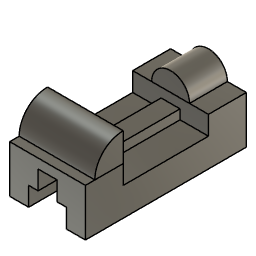
2 (Autodesk Fusion 360 design; units mm, degrees)
Autodesk Fusion 360 part; units mm, degrees
sketch "Sketch1" plane through (0, 0, 0) normal (0, 1, 0) x (1, 0, 0)
  line L0 (0, 0) -> (0, -50)
  line L1 (0, -50) -> (80, -50)
  line L2 (80, -50) -> (80, 0)
  line L3 (80, 0) -> (60, 0)
  line L4 (60, 0) -> (60, -20)
  line L5 (60, -20) -> (50, -20)
  line L6 (50, -20) -> (50, -40)
  line L7 (50, -40) -> (30, -40)
  line L8 (30, -40) -> (30, -20)
  line L9 (30, -20) -> (20, -20)
  line L10 (20, -20) -> (20, 0)
  line L11 (20, 0) -> (0, 0)
  dimension "d1" = 50
  constraint coincident L0.start L11.end
  constraint vertical L0
  constraint perpendicular L0 L1
  constraint perpendicular L1 L2
  constraint perpendicular L2 L3
  constraint perpendicular L3 L4
  constraint perpendicular L4 L5
  constraint perpendicular L3 L6
  constraint perpendicular L6 L7
  constraint perpendicular L7 L8
  constraint perpendicular L8 L9
  constraint perpendicular L9 L10
  constraint perpendicular L0 L11
  measures "d1" distance of L0.start L0.end
sketch "Sketch2" plane through (0, 0, 0) normal (0, 0, 1) x (1, 0, 0)
  line L0 (0, 0) -> (0, 170)
  line L1 (0, 170) -> (20, 170)
  line L2 (20, 170) -> (20, 0)
  line L3 (80, 0) -> (80, 170)
  line L4 (80, 170) -> (60, 170)
  line L5 (60, 170) -> (60, 0)
  dimension "d3" = 170
  constraint coincident L0.start origin
  constraint vertical L0
  constraint perpendicular L0 L1
  constraint perpendicular L1 L2
  constraint vertical L3
  constraint perpendicular L3 L4
  constraint perpendicular L4 L5
  measures "d3" distance of L0.start L0.end
sketch "Sketch3" plane through (0, 0, 0) normal (1, 0, 0) x (0, 1, 0)
  line L0 (0, 50) -> (10, 50)
  arc A0 (40, 80) -> (10, 50) centre (40, 50) ccw
  line L1 (40, 80) -> (40, 30)
  line L2 (40, 30) -> (130, 30)
  line L3 (130, 30) -> (130, 50)
  line L4 (130, 50) -> (170, 50)
  line L5 (170, 50) -> (170, 0)
  line L6 (130, 30) -> (170, 30)
  line L7 (10, 50) -> (40, 50)
  constraint horizontal L0
  constraint vertical L1
  constraint perpendicular L1 L2
  constraint perpendicular L2 L3
  constraint perpendicular L3 L4
  constraint perpendicular L4 L5
  constraint coincident L5 L6.end
  constraint perpendicular L5 L6
  constraint coincident A0.centre L7.end
  constraint perpendicular L1 L7
extrude "Extrude1" add sketch "Sketch1" along normal blind 40 makes body 1
sketch "Sketch5" plane through (0, 40, 0) normal (0, 1, 0) x (-1, 0, 0)
  line L0 (-20, 0) -> (0, 0)
  line L1 (0, 0) -> (0, 50)
  line L2 (0, 50) -> (-80, 50)
  line L3 (-80, 50) -> (-80, 0)
  line L4 (-80, 0) -> (-60, 0)
  line L5 (-60, 0) -> (-60, 20)
  line L6 (-60, 20) -> (-50, 20)
  line L7 (-50, 20) -> (-50, 40)
  line L8 (-50, 40) -> (-30, 40)
  line L9 (-30, 40) -> (-30, 20)
  line L10 (-30, 20) -> (-20, 20)
  line L11 (-20, 20) -> (-20, 0)
  line L12 (-80, 0) -> (-80, 30)
  line L13 (-80, 30) -> (-50, 30)
  line L14 (-50, 20) -> (-60, 20)
  line L15 (-60, 0) -> (-80, 0)
  line L16 (-20, 0) -> (-20, 20)
  line L17 (-30, 20) -> (-30, 30)
  line L18 (0, 30) -> (0, 0)
  line L19 (-30, 30) -> (0, 30)
  line L20 (0, 0) -> (-20, 0)
  line L21 (-50, 30) -> (-50, 40)
  line L22 (-30, 40) -> (-30, 30)
  line L23 (-50, 30) -> (-30, 30)
  constraint coincident L3.end L4.start
  constraint coincident L3 L12.end
  constraint perpendicular L4 L12
  constraint midpoint L7 L13.end
  constraint perpendicular L7 L13
  constraint coincident L6.end L7.start
  constraint coincident L5.end L6.start
  constraint coincident L4.end L5.start
  constraint coincident L0.start L11.end
  constraint coincident L10.end L11.start
  constraint coincident L9.end L10.start
  constraint midpoint L9 L17.end
  constraint coincident L1 L18.start
  constraint coincident L0.end L1.start
  constraint perpendicular L0 L18
  constraint perpendicular L1 L19
  constraint coincident L7.end L8.start
  constraint coincident L8.end L9.start
extrude "Extrude2" add sketch "Sketch5" along normal blind 130 contours L3 L4 L5 L6 L7 L12 L13 L14 L15 bodies 1
extrude "Extrude3" add sketch "Sketch5" along normal blind 130 contours L0 L1 L9 L10 L11 L16 L17 L18 L19 L20 bodies 1
extrude "Extrude4" add sketch "Sketch5" along normal blind 90 separate body contours L7 L8 L9 L21 L22 L23 makes body 2
extrude "Extrude5" add sketch "Sketch3" along normal blind 80 contours L3 L4 L5 L6 bodies 1 2
extrude "Extrude6" add sketch "Sketch3" along normal blind 80 separate body contours A0 L1 L7 makes body 3
sketch "Sketch6" plane through (0, 170, 0) normal (0, 1, 0) x (-1, 0, 0)
  line L0 (-30, 20) -> (-20, 20)
  line L1 (-20, 20) -> (-20, 0)
  line L2 (-20, 0) -> (0, 0)
  line L3 (0, 0) -> (0, 50)
  line L4 (0, 50) -> (-80, 50)
  line L5 (-80, 50) -> (-80, 0)
  line L6 (-80, 0) -> (-60, 0)
  line L7 (-60, 0) -> (-60, 20)
  line L8 (-60, 20) -> (-50, 20)
  line L9 (-50, 20) -> (-50, 30)
  line L10 (-50, 30) -> (-30, 30)
  line L11 (-30, 30) -> (-30, 20)
  arc A0 (-20, 50) -> (-60, 50) centre (-40, 50) ccw
  line L12 (-60, 50) -> (-20, 50)
  constraint coincident L4 A0.start
  constraint coincident L4 A0.end
  constraint midpoint L4 A0.centre
extrude "Extrude7" add sketch "Sketch6" against normal blind 40 separate body contours L4 A0 L12 makes body 4
